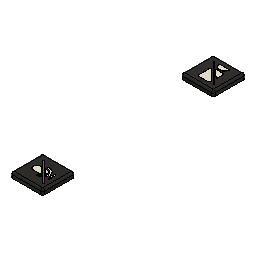
ZoomMuter_Keys_v11 (Autodesk Fusion 360 design; units mm, degrees)
Autodesk Fusion 360 part; units mm, degrees
sketch "Sketch1" plane through (0, 0, 0) normal (0, 1, 0) x (1, 0, 0)
  line L0 (0.615, 2.385) -> (-0.615, 2.385)
  line L1 (-0.615, -2.385) -> (0.615, -2.385)
  line L2 (0.615, 2.385) -> (-0.615, -2.385) construction
  line L3 (-0.615, 2.385) -> (0.615, -2.385) construction
  line L4 (-2.385, 0.59) -> (-2.385, -0.59)
  line L5 (2.385, -0.59) -> (2.385, 0.59)
  line L6 (2.385, 0.59) -> (-2.385, -0.59) construction
  line L7 (-2.385, 0.59) -> (2.385, -0.59) construction
  line L8 (2.385, 0.59) -> (0.615, 0.59)
  line L9 (-0.615, 0.59) -> (-2.385, 0.59)
  line L10 (0.615, -2.385) -> (0.615, -0.59)
  line L11 (0.615, 0.59) -> (0.615, 2.385)
  line L12 (-2.385, -0.59) -> (-0.615, -0.59)
  line L13 (0.615, -0.59) -> (2.385, -0.59)
  line L14 (-0.615, 2.385) -> (-0.615, 0.59)
  line L15 (-0.615, -0.59) -> (-0.615, -2.385)
  line L16 (-2.585, 0.79) -> (-2.585, -0.79)
  line L17 (-2.585, -0.79) -> (-0.815, -0.79)
  line L18 (-0.815, -0.79) -> (-0.815, -2.585)
  line L19 (-0.815, -2.585) -> (0.815, -2.585)
  line L20 (0.815, -2.585) -> (0.815, -0.79)
  line L21 (0.815, -0.79) -> (2.585, -0.79)
  line L22 (2.585, -0.79) -> (2.585, 0.79)
  line L23 (2.585, 0.79) -> (0.815, 0.79)
  line L24 (0.815, 0.79) -> (0.815, 2.585)
  line L25 (0.815, 2.585) -> (-0.815, 2.585)
  line L26 (-0.815, 2.585) -> (-0.815, 0.79)
  line L27 (-0.815, 0.79) -> (-2.585, 0.79)
  line L28 (12.5, -12.5) -> (-12.5, -12.5)
  line L29 (-12.5, -12.5) -> (-12.5, 12.5)
  line L30 (-12.5, 12.5) -> (12.5, 12.5)
  line L31 (12.5, 12.5) -> (12.5, -12.5)
  line L32 (12.5, -12.5) -> (-12.5, 12.5) construction
  line L33 (-12.5, -12.5) -> (12.5, 12.5) construction
  line L34 (4.0693, 4.0693) -> (-4.0693, 4.0693)
  line L35 (-4.0693, 4.0693) -> (-4.0693, -4.0693)
  line L36 (-4.0693, -4.0693) -> (4.0693, -4.0693)
  line L37 (4.0693, -4.0693) -> (4.0693, 4.0693)
  line L38 (4.0693, 4.0693) -> (-4.0693, -4.0693) construction
  line L39 (-4.0693, 4.0693) -> (4.0693, -4.0693) construction
  dimension "d1" = 4.77
  dimension "d2" = 1.23
  dimension "d3" = 4.77
  dimension "d4" = 1.18
  dimension "d5" = 0.2
  dimension "d6" = 25
  dimension "d7" = 25
  constraint perpendicular L0 L14
  constraint parallel L0 L1
  constraint parallel L10 L14
  constraint horizontal L0
  constraint coincident L2 origin
  constraint coincident L3 origin
  constraint perpendicular L4 L8
  constraint parallel L8 L12
  constraint parallel L4 L5
  constraint horizontal L8
  constraint coincident L6 origin
  constraint coincident L7 origin
  constraint collinear L8 L9
  constraint coincident L8.end L10
  constraint collinear L10 L11
  constraint coincident L10.end L12
  constraint collinear L12 L13
  constraint coincident L12.end L14
  constraint collinear L14 L15
  constraint perpendicular L28 L29
  constraint parallel L28 L30
  constraint parallel L29 L31
  constraint horizontal L28
  constraint coincident L32 origin
  constraint coincident L33 origin
  constraint perpendicular L34 L35
  constraint parallel L34 L36
  constraint parallel L35 L37
  constraint horizontal L34
  constraint coincident L33 L34.start
  constraint coincident L38 origin
  constraint coincident L39 origin
  measures "d1" distance of L0.end L1.start
  measures "d2" distance of L1.start L1.end
  measures "d3" distance of L4.end L5.start
  measures "d4" distance of L4.start L4.end
  measures "d6" distance of L29.end L30.end
  measures "d7" distance of L28.end L29.end
extrude "Extrude1" add sketch "Sketch1" along normal blind 4 contours L0 L1 L4 L5 L8 L9 L10 L11 L12 L13 L14 L15 | L16 L17 L18 L19 L20 L21 L22 L23 L24 L25 L26 L27 | L28 L29 L30 L31 | L34 L35 L36 L37 makes body 1
extrude "Extrude2" add sketch "Sketch1" against normal blind 4 contours L34 L35 L36 L37 bodies 1
fillet "Fillet1" radius 1.5 8 edges at (-12.5, 2, -12.5) (-12.5, 4, 0) (-12.5, 2, 12.5) (0, 4, 12.5) (12.5, 2, 12.5) (12.5, 4, 0) (12.5, 2, -12.5) (0, 4, -12.5) on bodies 1
sketch "Sketch2" plane through (0, 4, 0) normal (0, 1, 0) x (-1, 0, 0)
  line L0 (11, 11) -> (-11, 11)
  line L1 (-11, 11) -> (-11, -11)
  line L2 (-11, -11) -> (11, -11)
  line L3 (11, -11) -> (11, 11)
  line L4 (4.5487, 2.6853) -> (-1.0379, 2.6853)
  line L5 (-7.7641, 2.356) -> (-7.7641, -2.3937)
  line L6 (-6.7917, 0.6578) -> (-5.2066, 0.6578)
  line L7 (-6.7917, -0.6161) -> (-5.212, -0.6161)
  line L8 (-7.7928, 8.1709) -> (7.6836, -7.2774)
  line L9 (7.6836, -7.2774) -> (6.9848, -7.9775)
  line L10 (6.9848, -7.9775) -> (-8.4917, 7.4708)
  line L11 (-8.4917, 7.4708) -> (-7.7928, 8.1709)
  arc A0 (-7.7641, -2.3937) -> (-6.7917, -2.3937) centre (-7.2779, -2.3937) ccw
  arc A1 (-6.7917, 2.356) -> (-7.7641, 2.356) centre (-7.2779, 2.356) ccw
  line L12 (-6.7917, -2.3937) -> (-6.7917, -0.6161)
  line L13 (-6.7917, 0.6578) -> (-6.7917, 2.356)
  arc A2 (-5.212, -0.6161) -> (-0.0927, -4.7847) centre (-0.4527, 0.0008) ccw
  line L14 (-0.6807, -2.5882) -> (0.7007, -2.5882)
  arc A3 (4.5487, -2.5882) -> (4.5487, 2.6853) centre (4.5487, 0.0486) ccw
  line L15 (3.7687, -2.4701) -> (3.8869, -2.5882)
  line L16 (0.4742, -2.5882) -> (0.7007, -2.5882)
  line L17 (3.8869, -2.5882) -> (4.5487, -2.5882)
  arc A4 (-1.0379, 2.6853) -> (-1.3375, 2.6268) centre (-0.6807, 0.0607) ccw
  arc A5 (-3.0792, 1.1848) -> (-0.6807, -2.5882) centre (-0.6807, 0.0607) ccw
  line L18 (0.7007, -2.5882) -> (-3.0792, 1.1848)
  line L19 (-3.6969, 1.8014) -> (-4.4909, 2.594)
  line L20 (-1.3375, 2.6268) -> (3.7687, -2.4701)
  arc A6 (-4.4909, 2.594) -> (-5.2066, 0.6578) centre (-0.4527, 0.0008) ccw
  arc A7 (-3.6969, 1.8014) -> (-0.1521, -3.6624) centre (-0.3627, 0.0827) ccw
  arc A8 (-0.1464, 4.7901) -> (-2.8638, 4.1503) centre (-0.4527, 0.0008) ccw
  arc A9 (-0.1981, 3.8302) -> (-2.1127, 3.4006) centre (-0.3627, 0.0827) ccw
  line L21 (-0.8261, 2.1163) -> (-1.3375, 2.6268)
  line L22 (-2.1127, 3.4006) -> (-2.8638, 4.1503)
  arc A10 (-0.0927, -4.7847) -> (-0.177, -3.6638) centre (-0.1349, -4.2242) ccw
  arc A11 (-0.1981, 3.8302) -> (-0.1559, 4.7907) centre (-0.177, 4.3105) ccw
  constraint horizontal L4
  constraint horizontal L14
  constraint tangent L14 A4
  constraint tangent L14 A3
  constraint tangent A2 A10
  constraint vertical L5
  constraint vertical L12
  constraint horizontal L6
  constraint coincident L6.start L12
  constraint horizontal L7
  constraint perpendicular L8 L9
  constraint parallel L8 L10
  constraint parallel L9 L11
  constraint collinear L12 L13
  constraint coincident L19.end A2
  constraint coincident A7.end A10
  constraint coincident L14 L16.start
  constraint tangent A3 L16
  constraint horizontal L16
  constraint coincident L15.end L16
  constraint collinear L16 L17
  constraint concentric A4 A5
  constraint coincident L19.start A9
  constraint collinear L18 L19
  constraint concentric A6 A8
  constraint concentric A7 A9
  constraint coincident L20 L21.start
  constraint parallel L20 L21
  constraint coincident A9.end L21
  constraint collinear L21 L22
  constraint coincident A7 A10.end
  constraint coincident A8 A11.end
copy_body "CopyPasteBodies1" bodies 1 makes body 2
move_body "Move1" bodies 2 to x (1, 0, 0) y (0, 1, 0) z (0, 0, 1) at (0, 0, -131.6421)
sketch "Sketch3" plane through (0, 4, 0) normal (0, 1, 0) x (-1, 0, 0)
  line L0 (11, -120.6421) -> (-11, -120.6421)
  line L1 (-11, -120.6421) -> (-11, -142.6421)
  line L2 (-11, -142.6421) -> (11, -142.6421)
  line L3 (11, -142.6421) -> (11, -120.6421)
  line L4 (1.3975, -135.1379) -> (-5.0154, -128.7367)
  line L5 (7.6836, -139.1316) -> (6.9848, -139.8317)
  line L6 (-4.8471, -125.7242) -> (3.524, -134.0801)
  line L7 (-8.4917, -124.3834) -> (-7.7928, -123.6833)
  line L8 (6.9848, -139.8317) -> (-8.4917, -124.3834)
  line L9 (-7.7928, -123.6833) -> (7.6836, -139.1316)
  line L10 (4.3817, -125.014) -> (4.3817, -125.5201)
  line L11 (4.3817, -125.5201) -> (4.3817, -132.5328)
  line L12 (-5.0154, -128.7367) -> (-5.0154, -134.1414)
  line L13 (1.3975, -135.1379) -> (-3.9143, -135.1379)
  line L14 (3.3153, -123.7669) -> (-3.2275, -123.7669)
  line L15 (1.5802, -136.3826) -> (-2.2696, -136.3826)
  line L16 (-2.2696, -136.3826) -> (-4.3481, -138.9672)
  line L17 (1.5802, -136.3826) -> (3.5503, -138.9672)
  line L18 (3.0623, -139.9432) -> (-3.7155, -139.9432)
  arc A0 (3.0623, -139.9432) -> (3.5503, -138.9672) centre (3.0623, -139.3332) ccw
  arc A1 (-4.3481, -138.9672) -> (-3.7155, -139.9432) centre (-3.7155, -139.2502) ccw
  arc A2 (-5.0154, -134.1414) -> (-3.9143, -135.1379) centre (-3.9143, -134.0314) ccw
  line L19 (-5.0154, -129.1174) -> (-5.0154, -128.7367)
  arc A3 (-3.2275, -123.7669) -> (-4.8471, -125.7242) centre (-2.8675, -125.7135) ccw
  arc A4 (4.3817, -125.014) -> (3.3153, -123.7669) centre (3.1193, -125.014) ccw
  arc A5 (3.524, -134.0801) -> (4.3817, -132.5328) centre (2.5573, -132.5328) ccw
  point P0 (0, -131.8542)
  dimension "d14" = 0.6252
  dimension "d15" = 0.6366
  dimension "d16" = 0.9892
  constraint perpendicular L5 L9
  constraint parallel L8 L9
  constraint parallel L5 L7
  constraint parallel L6 L9
  constraint parallel L4 L8
  constraint vertical L10
  constraint parallel L10 L11
  constraint vertical L12
  constraint horizontal L13
  constraint horizontal L14
  constraint parallel L0 L15
  constraint horizontal L18
  constraint tangent L18 A0
  constraint tangent L18 A1
  constraint tangent L13 A2
  constraint coincident L12 L19.start
  constraint tangent L10 A4
  constraint tangent L11 A5
  measures "d14" distance of L4 L8
  measures "d15" distance of L6 L9
  measures "d16" distance of L8 L9
extrude "Extrude3" add sketch "Sketch2" sketch "Sketch3" against normal blind 0.2 separate body contours L4 A3 L15 L17 A4 L20 L21 | L5 L6 L7 A0 A1 L12 L13 A2 L19 A6 A7 A10 | L8 L9 L10 L11 | L14 L16 A5 L18 | A8 A9 L22 A11 of sketch 2 contours L4 L12 L13 A2 L19 | L5 L7 L8 L9 | L6 L10 L11 L14 A3 A4 A5 | L15 L16 L17 L18 A0 A1 makes body 3 at (2.8669, 4, -129.0661) makes body 4 at (2.5107, 4, -133.0042) makes body 5 at (2.4013, 4, 4.0035) makes body 6 at (-2.4659, 4, 0.9275) makes body 7 at (2.8669, 4, 2.7881) makes body 8 at (2.2854, 4, -0.8098) makes body 9 at (7.4399, 4, -0.2179) makes body 10 at (-1.3054, 4, -127.757) makes body 11 at (-0.309, 4, -138.7564)
extrude "Extrude4" cut sketch "Sketch2" sketch "Sketch3" against normal blind 0.2 contours L4 A3 L15 L17 A4 L20 L21 | L5 L6 L7 A0 A1 L12 L13 A2 L19 A6 A7 A10 | L8 L9 L10 L11 | L14 L16 A5 L18 | A8 A9 L22 A11 of sketch 2 contours L4 L12 L13 A2 L19 | L5 L7 L8 L9 | L6 L10 L11 L14 A3 A4 A5 | L15 L16 L17 L18 A0 A1 bodies 1 2
ref_plane "WorkPlane1" through (0, 0.215, 0) normal (0, -1, 0) x (-1, 0, 0)
split "Split1" [rolled back]
equation "d5 = tolerance"
equation "tolerance = 0.2 mm"
equation "d19 = -layer_height"
equation "d21 = -layer_height"
equation "layer_height = 0.2 mm"
named bodies: "MuteKey", "VideoKey", "VideoSlash", "VideoSymbol1", "MuteSymbol3", "MuteSymbol1", "MuteSlash", "MuteSymbol2", "MuteSymbol4", "VideoSymbol2", "VideoSymbol3"
